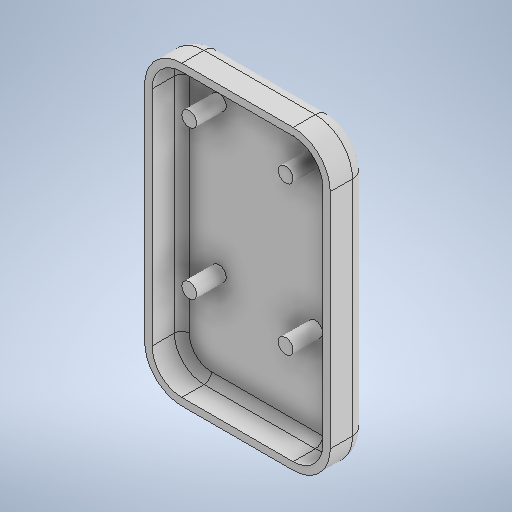
# Autodesk Inventor part: Carcaca-Baixa
Saved by Autodesk Inventor 2025 (Build 290162010, 162A)
## iProperties
Created: 2025-10-21
Part Number: Carcaca-Baixa
Material: Genérico
Document SubType Name: Modeling
Designer: 202321250026
Density: 1 g/cm^3
Appearance: Padrão
Author: 202321250026
Autodesk Inventor part; units mm, degrees
ref_plane "YZ Plane" through (0, 0, 0) normal (1, 0, 0) x (0, 1, 0)
ref_plane "XZ Plane" through (0, 0, 0) normal (0, 1, 0) x (-1, 0, 0)
ref_plane "XY Plane" through (0, 0, 0) normal (0, 0, 1) x (1, 0, 0)
sketch "Esboço1" plane through (0, 0, 0) normal (0, 0, 1) x (1, 0, 0)
  line L0 (-29.0921, 25.5754) -> (20.9079, 25.5754)
  line L1 (20.9079, 25.5754) -> (20.9079, -54.4246)
  line L2 (20.9079, -54.4246) -> (-29.0921, -54.4246)
  line L3 (-29.0921, -54.4246) -> (-29.0921, 25.5754)
  point P0 (0, 0)
  constraints: 8 end point, 2 parallel, 1 horizontal, 1 perpendicular
extrude "Extrusão1" add sketch "Esboço1" along normal blind 10
fillet "Arredondamento1" radius 10 4 edges at (-29.0921, 25.5754, 5) (20.9079, 25.5754, 5) (20.9079, -54.4246, 5) (-29.0921, -54.4246, 5)
fillet "Arredondamento2" radius 4 8 edges at (-26.1631, 22.6465, 0) (-29.0921, -14.4246, 0) (-26.1631, -51.4956, 0) (-4.0921, -54.4246, 0) (17.979, -51.4956, 0) (20.9079, -14.4246, 0) (17.979, 22.6465, 0) (-4.0921, 25.5754, 0)
shell "Casca1" thickness 2 removed faces 1 at (-12.4254, -4.4246, 10)
sketch "Esboço2" plane through (-19.0921, -50.4246, 2) normal (0, 0, 1) x (1, 0, 0)
  arc A0 (-8, 6) -> (0, -2) centre (0, 6) ccw projected
  line L0 (-8, 6) -> (-8, 66) projected
  arc A1 (0, 74) -> (-8, 66) centre (0, 66) ccw projected
  line L1 (0, 74) -> (30, 74) projected
  arc A2 (38, 66) -> (30, 74) centre (30, 66) ccw projected
  line L2 (38, 66) -> (38, 6) projected
  arc A3 (30, -2) -> (38, 6) centre (30, 6) ccw projected
  line L3 (30, -2) -> (0, -2) projected
  arc A4 (-10, 6) -> (0, -4) centre (0, 6) ccw projected
  line L4 (0, -4) -> (30, -4) projected
  arc A5 (30, -4) -> (40, 6) centre (30, 6) ccw projected
  line L5 (40, 6) -> (40, 66) projected
  arc A6 (40, 66) -> (30, 76) centre (30, 66) ccw projected
  line L6 (30, 76) -> (0, 76) projected
  arc A7 (0, 76) -> (-10, 66) centre (0, 66) ccw projected
  line L7 (-10, 66) -> (-10, 6) projected
  arc A8 (0, 72) -> (-6, 66) centre (0, 66) ccw projected
  circle A9 centre (2, 64) radius 2
  circle A10 centre (28, 64) radius 2
  circle A11 centre (2, 24) radius 2
  circle A12 centre (28, 24) radius 2
  point P0 (19.0921, 50.4246)
  dimension "d16" = 8
  dimension "d17" = 8
  dimension "d18" = 36
  dimension "d19" = 36
  dimension "d20" = 12
  dimension "d21" = 12
  constraints: 4 centre point
  measures "d16" distance edge to line of A9 L1
  measures "d17" distance edge to line of A10 L1
  measures "d20" distance from line of L7 A9.centre
  measures "d21" distance from line of L5 A10.centre
extrude "Extrusão2" add sketch "Esboço2" along normal up to surface (8 mm away) contours A9 | A10 | A11 | A12
equation "\"d17\" = d16"
equation "\"d19\" = d18"
